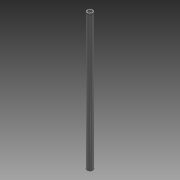
# Autodesk Inventor part: Fixture_Weight_Shaft-02
Saved by Autodesk Inventor 2015 (Build 190159000, 159)
## iProperties
Created: 2015-01-18
Part Number: Fixture_Weight_Shaft-02
Material: Stainless Steel
Document SubType Name: Modeling
Designer: Drew
Density: 8 g/cm^3
Appearance: Semi-Polished
Author: Drew
Autodesk Inventor part; units mm, degrees
ref_plane "YZ Plane" through (0, 0, 0) normal (1, 0, 0) x (0, 1, 0)
ref_plane "XZ Plane" through (0, 0, 0) normal (0, 1, 0) x (-1, 0, 0)
ref_plane "XY Plane" through (0, 0, 0) normal (0, 0, 1) x (1, 0, 0)
sketch "Sketch1" plane through (0, 0, 0) normal (0, 0, 1) x (1, 0, 0)
  line L0 (0, 0) -> (0, 149.606)
  line L1 (0, 149.606) -> (3.175, 149.606)
  line L2 (3.175, 149.606) -> (3.175, 148.59)
  line L3 (3.175, 148.59) -> (2.921, 148.59)
  line L4 (2.921, 148.59) -> (2.921, 147.828)
  line L5 (2.921, 147.828) -> (3.175, 147.828)
  line L6 (3.175, 147.828) -> (3.175, 0)
  line L7 (3.175, 0) -> (0, 0)
  dimension "d0" = 3.175
  dimension "d1" = 149.606
  dimension "d2" = 0.762
  dimension "d3" = 0.254
  dimension "d4" = 1.016
  constraints: 16 end point, 6 perpendicular, 2 point on line, 1 vertical
  measures "d0" distance of L0.end L1.end
  measures "d1" distance between parallel lines of L7 L1
  measures "d2" distance between parallel lines of L5 L3
  measures "d3" distance between parallel lines of L4 L2
  measures "d4" distance between parallel lines of L1 L3
revolve "Revolution1" add sketch "Sketch1" angle 360 about axis through (0, 0, 0) along (0, 1, 0)
sketch "Sketch2" plane through (0, 149.606, 0) normal (0, 1, 0) x (1, 0, 0)
  point P0 (0, 0)
  point P1 (0, 0)
  constraints: 1 coincident
hole "Hole1" at (0, 149.606, 0) direction (0, -1, 0) diameter 3.9624 depth 10.16 tip angle 118 thread size "10-32 UNF" class "2B" standard "ANSI Unified Screw Threads"
sketch "Sketch3" plane through (0, 0, 0) normal (0, -1, 0) x (1, 0, 0)
  point P0 (0, 0)
  point P1 (0, 0)
  constraints: 1 coincident
hole "Hole2" at (0, 0, 0) direction (0, 1, 0) diameter 3.302 depth 10.16 tip angle 118 thread size "8-32 UNC" class "2B" standard "ANSI Unified Screw Threads"
body "Solid1"
